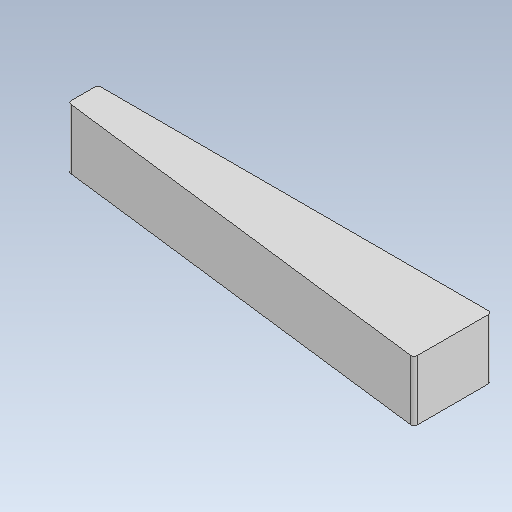
# Autodesk Inventor part: Wedge
Saved by Autodesk Inventor 2020 (Build 240168000, 168)
## iProperties
Created: 2020-03-08
Part Number: Wedge
Material: Generic
Document SubType Name: Modeling
Designer: Daniel Wikman
Density: 1 g/cm^3
Appearance: Default
Author: Daniel Wikman
Autodesk Inventor part; units mm, degrees
ref_plane "YZ Plane" through (0, 0, 0) normal (1, 0, 0) x (0, 1, 0)
ref_plane "XZ Plane" through (0, 0, 0) normal (0, 1, 0) x (-1, 0, 0)
ref_plane "XY Plane" through (0, 0, 0) normal (0, 0, 1) x (1, 0, 0)
sketch "Sketch1" plane through (0, 0, 0) normal (0, 1, 0) x (-1, 0, 0)
  line L0 (-2.4599, -13.6593) -> (-41.1266, -13.6593)
  arc A0 (-41.4599, -13.326) -> (-41.1266, -13.6593) centre (-41.1266, -13.326) ccw
  arc A1 (-2.4599, -13.6593) -> (-2.1266, -13.326) centre (-2.4599, -13.326) ccw
  line L1 (-2.1266, -13.326) -> (-2.1266, -10.9926)
  arc A2 (-2.1266, -10.9926) -> (-2.4599, -10.6593) centre (-2.4599, -10.9926) ccw
  line L2 (-2.4599, -10.6593) -> (-41.086, -5.9166)
  arc A3 (-41.086, -5.9166) -> (-41.4599, -6.2475) centre (-41.1266, -6.2475) ccw
  line L3 (-41.4599, -13.326) -> (-41.4599, -6.2475)
  point P0 (0, 0)
  dimension "d0" = 38.6667
  dimension "d1" = 0.6667
  dimension "d2" = 0.6667
  dimension "d4" = 0.6667
  dimension "d5" = 2.6667
  dimension "d6" = 7
  dimension "d7" = 0.6667
  dimension "d11" = 39.3333
  constraints: 9 point on circle, 8 end point, 6 tangent, 4 centre point, 2 vertical, 1 horizontal, 1 point on line
  measures "d0" distance of L0.start L0.end
  measures "d1" diameter of A0
  measures "d2" diameter of A1
  measures "d4" diameter of A2
  measures "d5" distance from line of A2.centre L0
  measures "d6" angle of L0 L2
  measures "d7" diameter of A3
  measures "d11" distance between parallel lines of L3 L1
extrude "Extrusion1" add sketch "Sketch1" along normal blind 6
body "Solid1"
